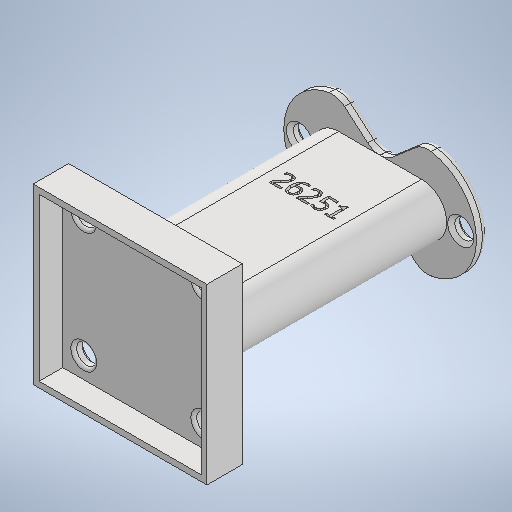
# Autodesk Inventor part: OTOSmount
Saved by Autodesk Inventor 2025.2 (Build 292293000, 293)
## iProperties
Created: 2025-01-03
Part Number: OTOSmount
Material: Generic
Document SubType Name: Modeling
Designer: dcfam
Density: 1 g/cm^3
Appearance: Default
Author: dcfam
Autodesk Inventor part; units mm, degrees
ref_plane "YZ Plane" through (0, 0, 0) normal (1, 0, 0) x (0, 1, 0)
ref_plane "XZ Plane" through (0, 0, 0) normal (0, 1, 0) x (-1, 0, 0)
ref_plane "XY Plane" through (0, 0, 0) normal (0, 0, 1) x (1, 0, 0)
sketch "Sketch1" plane through (0, 0, 0) normal (0, 0, 1) x (1, 0, 0)
  line L0 (-12.7, -12.7) -> (12.7, -12.7) construction
  line L1 (12.7, -12.7) -> (12.7, 12.7) construction
  line L2 (12.7, 12.7) -> (-12.7, 12.7) construction
  line L3 (-12.7, 12.7) -> (-12.7, -12.7) construction
  line L4 (-12.7, -12.7) -> (12.7, 12.7) construction
  line L5 (12.7, -12.7) -> (-12.7, 12.7) construction
  line L6 (14.7, -14.7) -> (-14.7, -14.7)
  line L7 (-14.7, -14.7) -> (-14.7, 14.7)
  line L8 (-14.7, 14.7) -> (14.7, 14.7)
  line L9 (14.7, 14.7) -> (14.7, -14.7)
  point P0 (0, 0)
  dimension "d0" = 25.4
  dimension "d1" = 25.4
  dimension "d2" = 2
  constraints: 20 end point, 4 parallel, 2 midpoint, 2 perpendicular, 1 horizontal, 3 other
  measures "d0" distance of L2.end L1.end
  measures "d1" distance of L1.end L0.end
  measures "d2" distance between parallel lines of L0 L6
extrude "Extrusion1" add sketch "Sketch1" along normal blind 2
sketch "Sketch2" plane through (0, 0, 2) normal (0, 0, 1) x (1, 0, 0)
  line L0 (-12.7, -12.7) -> (12.7, -12.7) construction
  line L1 (12.7, -12.7) -> (12.7, 12.7) construction
  line L2 (12.7, 12.7) -> (-12.7, 12.7) construction
  line L3 (-12.7, 12.7) -> (-12.7, -12.7) construction
  line L4 (-12.7, -12.7) -> (12.7, 12.7) construction
  line L5 (12.7, -12.7) -> (-12.7, 12.7) construction
  circle A0 centre (-10.16, 10.16) radius 1.675
  line L6 (0, 12.7) -> (0, -12.7) construction
  line L7 (-12.7, 0) -> (12.7, 0) construction
  circle A1 centre (10.16, 10.16) radius 1.675
  circle A2 centre (-10.16, -10.16) radius 1.675
  circle A3 centre (10.16, -10.16) radius 1.675
  point P0 (0, 0)
  dimension "d5" = 25.4
  dimension "d6" = 25.4
  dimension "d7" = 3.35
  dimension "d8" = 2.54
  dimension "d9" = 2.54
  constraints: 16 end point, 6 midpoint, 4 centre point, 3 symmetric about line, 2 parallel, 1 horizontal, 1 perpendicular, 3 other
  measures "d5" distance of L2.end L1.end
  measures "d6" distance of L1.end L0.end
  measures "d7" diameter of A0
  measures "d8" distance from line of L3 A0.centre
  measures "d9" distance from line of L2 A0.centre
extrude "Extrusion2" cut sketch "Sketch2" against normal blind 100
sketch "Sketch4" plane through (0, 0, 0) normal (0, 0, -1) x (-1, 0, 0)
  line L0 (-14.7, 14.7) -> (14.7, 14.7) construction
  line L1 (0, 14.7) -> (0, -14.7) construction
  line L2 (14.7, -14.7) -> (-14.7, -14.7) construction
  line L3 (-14.7, -14.7) -> (-14.7, 14.7) construction
  line L4 (-14.7, 0) -> (14.7, 0) construction
  line L5 (14.7, 14.7) -> (14.7, -14.7) construction
  line L6 (-12.7, -12.7) -> (12.7, -12.7) construction
  line L7 (12.7, -12.7) -> (12.7, 12.7) construction
  line L8 (12.7, 12.7) -> (-12.7, 12.7) construction
  line L9 (-12.7, 12.7) -> (-12.7, -12.7) construction
  line L10 (-12.7, -12.7) -> (12.7, 12.7) construction
  line L11 (12.7, -12.7) -> (-12.7, 12.7) construction
  line L12 (-7.021, 0) -> (7.021, 0) construction
  line L13 (-7.021, -4.254) -> (7.021, -4.254)
  line L14 (7.021, 4.254) -> (-7.021, 4.254)
  arc A0 (-7.021, 4.254) -> (-7.021, -4.254) centre (-7.021, 0) ccw
  arc A1 (7.021, -4.254) -> (7.021, 4.254) centre (7.021, 0) ccw
  point P0 (0, 0)
  dimension "d12" = 25.4
  dimension "d13" = 25.4
  constraints: 24 end point, 7 midpoint, 4 point on circle, 4 tangent, 3 parallel, 2 centre point, 1 horizontal, 1 perpendicular, 1 point on line
  measures "d12" distance of L8.end L7.end
  measures "d13" distance of L7.end L6.end
extrude "Extrusion3" add sketch "Sketch4" along normal blind 40
sketch "Sketch5" plane through (0, 0, -40) normal (0, 0, -1) x (-1, 0, 0)
  arc A0 (-7.021, 4.254) -> (-7.021, -4.254) centre (-7.021, 0) ccw projected
  arc A1 (7.021, -4.254) -> (7.021, 4.254) centre (7.021, 0) ccw projected
  arc A2 (7.021, -4.254) -> (7.021, 4.254) centre (7.021, 0) ccw projected
  line L0 (7.021, 4.254) -> (-7.021, 4.254) projected
  arc A3 (-7.021, 4.254) -> (-7.021, -4.254) centre (-7.021, 0) ccw projected
  line L1 (-7.021, -4.254) -> (7.021, -4.254) projected
  arc A4 (7.021, -9.254) -> (7.021, 9.254) centre (7.021, 0) ccw
  arc A5 (-7.021, 9.254) -> (-7.021, -9.254) centre (-7.021, 0) ccw
  circle A6 centre (13.6439, 0) radius 1.6
  line L2 (0, 9.254) -> (0, -9.254) construction
  circle A7 centre (-13.6439, 0) radius 1.6
  line L3 (-16.275, 0) -> (16.275, 0) construction
  line L4 (-7.021, -9.254) -> (-1.1973, -4.254)
  line L5 (-7.021, 9.254) -> (-1.1973, 4.254)
  line L6 (7.021, -9.254) -> (1.1973, -4.254)
  line L7 (7.021, 9.254) -> (1.1973, 4.254)
  point P0 (0, 0)
  point P1 (-1.1973, 4.254)
  point P2 (1.1973, 4.254)
  point P3 (1.1973, -4.254)
  dimension "d17" = 3.2
  constraints: 12 end point, 6 point on circle, 4 centre point, 4 symmetric about line, 1 point on line, 1 other
  measures "d17" diameter of A6
extrude "Extrusion4" add sketch "Sketch5" against normal blind 2
fillet "Fillet1" radius 3.175 8 edges at (-7.021, -9.254, -39) (7.021, -9.254, -39) (7.021, 9.254, -39) (-7.021, 9.254, -39) (1.1973, 4.254, -39) (-1.1973, 4.254, -39) (-1.1973, -4.254, -39) (1.1973, -4.254, -39)
chamfer "Chamfer1" distance 0.6 angle 45 4 edges at (-12.0439, 0, -38) (-12.0439, 0, -40) (15.2439, 0, -38) (15.2439, 0, -40)
fillet "Fillet2" radius 3.175 4 edges at (11.275, 0, 0) (0, 4.254, 0) (-11.275, 0, 0) (0, -4.254, 0)
chamfer "Chamfer2" distance 0.6 angle 45 4 edges at (-11.835, -10.16, 0) (8.485, -10.16, 0) (-11.835, 10.16, 0) (8.485, 10.16, 0)
sketch "Sketch7" plane through (0, 0, 2) normal (0, 0, 1) x (1, 0, 0)
  circle A0 centre (-10.16, 10.16) radius 1.675 projected
  circle A1 centre (10.16, -10.16) radius 1.675 projected
  circle A2 centre (-10.16, -10.16) radius 1.675 projected
  circle A3 centre (10.16, 10.16) radius 1.675 projected
  line L0 (14.7, 14.7) -> (-14.7, 14.7) projected
  line L1 (-14.7, 14.7) -> (-14.7, -14.7) projected
  line L2 (-14.7, -14.7) -> (14.7, -14.7) projected
  line L3 (14.7, -14.7) -> (14.7, 14.7) projected
  line L4 (12.7, 12.7) -> (-12.7, 12.7) construction
  line L5 (-12.7, 12.7) -> (-12.7, -12.7) construction
  line L6 (-12.7, -12.7) -> (12.7, -12.7) construction
  line L7 (12.7, -12.7) -> (12.7, 12.7) construction
  line L8 (12.7, 12.7) -> (-12.7, -12.7) construction
  line L9 (-12.7, 12.7) -> (12.7, -12.7) construction
  line L10 (13.7, -13.7) -> (-13.7, -13.7)
  line L11 (-13.7, -13.7) -> (-13.7, 13.7)
  line L12 (-13.7, 13.7) -> (13.7, 13.7)
  line L13 (13.7, 13.7) -> (13.7, -13.7)
  point P0 (0, 0)
  dimension "d28" = 25.4
  dimension "d29" = 25.4
  dimension "d30" = 1
  constraints: 20 end point, 2 midpoint, 2 parallel, 1 horizontal, 1 perpendicular, 3 other
  measures "d28" distance of L6.end L5.end
  measures "d29" distance of L5.end L4.end
  measures "d30" distance between parallel lines of L2 L10
extrude "Extrusion5" add sketch "Sketch7" along normal blind 4 contours L3 L2 L1 L0
sketch "Sketch9" plane through (1.1973, 4.254, -38) normal (0, 1, 0) x (1, 0, 0)
  line L0 (-6.838, -10.2364) -> (4.4434, -10.2364) construction
  line L1 (4.4434, -10.2364) -> (4.4434, -14.3898) construction
  line L2 (4.4434, -14.3898) -> (-6.838, -14.3898) construction
  line L3 (-6.838, -14.3898) -> (-6.838, -10.2364) construction
  line L4 (-6.838, -10.2364) -> (4.4434, -14.3898)
  line L5 (4.4434, -10.2364) -> (-6.838, -14.3898)
  line L6 (5.8237, -34.825) -> (-8.2183, -34.825) construction
  line L7 (5.8237, -34.825) -> (5.8237, 0) construction
  line L8 (5.8237, 0) -> (-1.176, 0) construction
  line L9 (-1.2186, 2) -> (-1.176, 2) construction
  line L10 (-1.2186, 0) -> (-8.2183, 0) construction
  line L11 (-8.2183, -34.825) -> (-8.2183, 0) construction
  line L12 (-1.1973, 2) -> (-1.1973, -34.825) construction
  line L13 (-1.176, 2) -> (-1.176, 0) projected
  line L14 (-1.2186, 0) -> (-1.2186, 2) projected
  line L15 (-4.736, -13.3487) -> (-6.6157, -13.3487)
  line L16 (-6.6157, -13.3487) -> (-6.6157, -12.9164)
  spline S0 degree 2 poles (-6.6157, -12.9164) (-6.4132, -12.7262) (-6.0525, -12.373) (-5.8796, -12.1828) knots 0 0 0 1 2 2 2
  spline S1 degree 2 poles (-5.8796, -12.1828) (-5.5314, -11.8) (-5.277, -11.3405) (-5.277, -11.096) knots 0 0 0 1 2 2 2
  spline S2 degree 2 poles (-5.277, -11.096) (-5.277, -10.9676) (-5.356, -10.7749) (-5.4276, -10.7132) knots 0 0 0 1 2 2 2
  spline S3 degree 2 poles (-5.4276, -10.7132) (-5.4993, -10.6514) (-5.687, -10.5897) (-5.8006, -10.5897) knots 0 0 0 1 2 2 2
  spline S4 degree 2 poles (-5.8006, -10.5897) (-5.9093, -10.5897) (-6.1316, -10.644) (-6.2329, -10.686) knots 0 0 0 1 2 2 2
  spline S5 degree 2 poles (-6.2329, -10.686) (-6.3193, -10.7206) (-6.4799, -10.8194) (-6.5293, -10.8539) knots 0 0 0 1 2 2 2
  line L17 (-6.5293, -10.8539) -> (-6.5515, -10.8539)
  line L18 (-6.5515, -10.8539) -> (-6.5515, -10.4192)
  spline S6 degree 2 poles (-6.5515, -10.4192) (-6.4255, -10.3575) (-5.9735, -10.2364) (-5.771, -10.2364) knots 0 0 0 1 2 2 2
  spline S7 degree 2 poles (-5.771, -10.2364) (-5.3436, -10.2364) (-4.862, -10.6885) (-4.862, -11.0738) knots 0 0 0 1 2 2 2
  spline S8 degree 2 poles (-4.862, -11.0738) (-4.862, -11.2541) (-4.946, -11.5554) (-5.0201, -11.6839) knots 0 0 0 1 2 2 2
  spline S9 degree 2 poles (-5.0201, -11.6839) (-5.0942, -11.8172) (-5.3091, -12.0791) (-5.4276, -12.205) knots 0 0 0 1 2 2 2
  spline S10 degree 2 poles (-5.4276, -12.205) (-5.6203, -12.415) (-6.0921, -12.8645) (-6.2329, -12.9954) knots 0 0 0 1 2 2 2
  line L19 (-6.2329, -12.9954) -> (-4.736, -12.9954)
  line L20 (-4.736, -12.9954) -> (-4.736, -13.3487)
  spline S11 degree 2 poles (-2.4019, -12.3607) (-2.4019, -12.5953) (-2.5575, -12.993) (-2.6884, -13.1264) knots 0 0 0 1 2 2 2
  spline S12 degree 2 poles (-2.6884, -13.1264) (-2.8242, -13.2671) (-3.1651, -13.4129) (-3.3701, -13.4129) knots 0 0 0 1 2 2 2
  spline S13 degree 2 poles (-3.3701, -13.4129) (-3.5751, -13.4129) (-3.9135, -13.2746) (-4.0419, -13.1362) knots 0 0 0 1 2 2 2
  spline S14 degree 2 poles (-4.0419, -13.1362) (-4.2, -12.9707) (-4.3779, -12.415) (-4.3779, -12.0099) knots 0 0 0 1 2 2 2
  spline S15 degree 2 poles (-4.3779, -12.0099) (-4.3779, -11.6122) (-4.2148, -10.9725) (-4.0444, -10.7354) knots 0 0 0 1 2 2 2
  spline S16 degree 2 poles (-4.0444, -10.7354) (-3.8789, -10.5032) (-3.3553, -10.2438) (-3.0119, -10.2438) knots 0 0 0 1 2 2 2
  spline S17 degree 2 poles (-3.0119, -10.2438) (-2.9107, -10.2438) (-2.7328, -10.2636) (-2.6661, -10.2858) knots 0 0 0 1 2 2 2
  line L21 (-2.6661, -10.2858) -> (-2.6661, -10.6786)
  line L22 (-2.6661, -10.6786) -> (-2.6834, -10.6786)
  spline S18 degree 2 poles (-2.6834, -10.6786) (-2.7402, -10.6489) (-2.9477, -10.5971) (-3.0663, -10.5971) knots 0 0 0 1 2 2 2
  spline S19 degree 2 poles (-3.0663, -10.5971) (-3.4467, -10.5971) (-3.9135, -11.1108) (-3.958, -11.6147) knots 0 0 0 1 2 2 2
  spline S20 degree 2 poles (-3.958, -11.6147) (-3.8122, -11.5134) (-3.506, -11.4023) (-3.3232, -11.4023) knots 0 0 0 1 2 2 2
  spline S21 degree 2 poles (-3.3232, -11.4023) (-3.1453, -11.4023) (-2.8786, -11.4739) (-2.7328, -11.5826) knots 0 0 0 1 2 2 2
  spline S22 degree 2 poles (-2.7328, -11.5826) (-2.5649, -11.7086) (-2.4019, -12.0988) (-2.4019, -12.3607) knots 0 0 0 1 2 2 2
  spline S23 degree 2 poles (-2.8168, -12.3779) (-2.8168, -12.1902) (-2.9156, -11.9358) (-3.0243, -11.8469) knots 0 0 0 1 2 2 2
  spline S24 degree 2 poles (-3.0243, -11.8469) (-3.1058, -11.7827) (-3.3084, -11.7407) (-3.4146, -11.7407) knots 0 0 0 1 2 2 2
  spline S25 degree 2 poles (-3.4146, -11.7407) (-3.5578, -11.7407) (-3.8271, -11.8271) (-3.958, -11.9086) knots 0 0 0 1 2 2 2
  spline S26 degree 2 poles (-3.958, -11.9086) (-3.9604, -11.9531) (-3.9654, -12.0371) (-3.9654, -12.1013) knots 0 0 0 1 2 2 2
  spline S27 degree 2 poles (-3.9654, -12.1013) (-3.9654, -12.4175) (-3.8419, -12.8053) (-3.748, -12.9065) knots 0 0 0 1 2 2 2
  spline S28 degree 2 poles (-3.748, -12.9065) (-3.6616, -13.0029) (-3.4738, -13.0794) (-3.3676, -13.0794) knots 0 0 0 1 2 2 2
  spline S29 degree 2 poles (-3.3676, -13.0794) (-3.1206, -13.0794) (-2.8168, -12.7287) (-2.8168, -12.3779) knots 0 0 0 1 2 2 2
  line L23 (-0.1616, -13.3487) -> (-2.0412, -13.3487)
  line L24 (-2.0412, -13.3487) -> (-2.0412, -12.9164)
  spline S30 degree 2 poles (-2.0412, -12.9164) (-1.8387, -12.7262) (-1.4781, -12.373) (-1.3052, -12.1828) knots 0 0 0 1 2 2 2
  spline S31 degree 2 poles (-1.3052, -12.1828) (-0.9569, -11.8) (-0.7025, -11.3405) (-0.7025, -11.096) knots 0 0 0 1 2 2 2
  spline S32 degree 2 poles (-0.7025, -11.096) (-0.7025, -10.9676) (-0.7815, -10.7749) (-0.8532, -10.7132) knots 0 0 0 1 2 2 2
  spline S33 degree 2 poles (-0.8532, -10.7132) (-0.9248, -10.6514) (-1.1125, -10.5897) (-1.2261, -10.5897) knots 0 0 0 1 2 2 2
  spline S34 degree 2 poles (-1.2261, -10.5897) (-1.3348, -10.5897) (-1.5571, -10.644) (-1.6584, -10.686) knots 0 0 0 1 2 2 2
  spline S35 degree 2 poles (-1.6584, -10.686) (-1.7448, -10.7206) (-1.9054, -10.8194) (-1.9548, -10.8539) knots 0 0 0 1 2 2 2
  line L25 (-1.9548, -10.8539) -> (-1.977, -10.8539)
  line L26 (-1.977, -10.8539) -> (-1.977, -10.4192)
  spline S36 degree 2 poles (-1.977, -10.4192) (-1.851, -10.3575) (-1.399, -10.2364) (-1.1965, -10.2364) knots 0 0 0 1 2 2 2
  spline S37 degree 2 poles (-1.1965, -10.2364) (-0.7692, -10.2364) (-0.2875, -10.6885) (-0.2875, -11.0738) knots 0 0 0 1 2 2 2
  spline S38 degree 2 poles (-0.2875, -11.0738) (-0.2875, -11.2541) (-0.3715, -11.5554) (-0.4456, -11.6839) knots 0 0 0 1 2 2 2
  spline S39 degree 2 poles (-0.4456, -11.6839) (-0.5197, -11.8172) (-0.7346, -12.0791) (-0.8532, -12.205) knots 0 0 0 1 2 2 2
  spline S40 degree 2 poles (-0.8532, -12.205) (-1.0458, -12.415) (-1.5176, -12.8645) (-1.6584, -12.9954) knots 0 0 0 1 2 2 2
  line L27 (-1.6584, -12.9954) -> (-0.1616, -12.9954)
  line L28 (-0.1616, -12.9954) -> (-0.1616, -13.3487)
  spline S41 degree 2 poles (2.0936, -12.3804) (2.0936, -12.6002) (1.9528, -12.9757) (1.8243, -13.114) knots 0 0 0 1 2 2 2
  spline S42 degree 2 poles (1.8243, -13.114) (1.6959, -13.2523) (1.313, -13.4129) (1.0759, -13.4129) knots 0 0 0 1 2 2 2
  spline S43 degree 2 poles (1.0759, -13.4129) (0.8586, -13.4129) (0.4337, -13.3165) (0.2781, -13.24) knots 0 0 0 1 2 2 2
  line L29 (0.2781, -13.24) -> (0.2781, -12.8077)
  line L30 (0.2781, -12.8077) -> (0.3078, -12.8077)
  spline S44 degree 2 poles (0.3078, -12.8077) (0.3547, -12.8423) (0.5301, -12.9312) (0.6363, -12.9707) knots 0 0 0 1 2 2 2
  spline S45 degree 2 poles (0.6363, -12.9707) (0.7573, -13.0127) (0.9574, -13.0597) (1.0833, -13.0597) knots 0 0 0 1 2 2 2
  spline S46 degree 2 poles (1.0833, -13.0597) (1.2068, -13.0597) (1.439, -12.9707) (1.523, -12.8744) knots 0 0 0 1 2 2 2
  spline S47 degree 2 poles (1.523, -12.8744) (1.5996, -12.783) (1.6786, -12.541) (1.6786, -12.3779) knots 0 0 0 1 2 2 2
  spline S48 degree 2 poles (1.6786, -12.3779) (1.6786, -12.2149) (1.5897, -12.0074) (1.5057, -11.9383) knots 0 0 0 1 2 2 2
  spline S49 degree 2 poles (1.5057, -11.9383) (1.4193, -11.8617) (1.1624, -11.7975) (1.0068, -11.7975) knots 0 0 0 1 2 2 2
  spline S50 degree 2 poles (1.0068, -11.7975) (0.8388, -11.7975) (0.5054, -11.8494) (0.4041, -11.8716) knots 0 0 0 1 2 2 2
  line L31 (0.4041, -11.8716) -> (0.4041, -10.3007)
  line L32 (0.4041, -10.3007) -> (2.0763, -10.3007)
  line L33 (2.0763, -10.3007) -> (2.0763, -10.6588)
  line L34 (2.0763, -10.6588) -> (0.7968, -10.6588)
  line L35 (0.7968, -10.6588) -> (0.7968, -11.4714)
  spline S51 degree 2 poles (0.7968, -11.4714) (0.8709, -11.4616) (1.0142, -11.4542) (1.0735, -11.4542) knots 0 0 0 1 2 2 2
  spline S52 degree 2 poles (1.0735, -11.4542) (1.3081, -11.4542) (1.6317, -11.5307) (1.7799, -11.6443) knots 0 0 0 1 2 2 2
  spline S53 degree 2 poles (1.7799, -11.6443) (1.9306, -11.758) (2.0936, -12.1038) (2.0936, -12.3804) knots 0 0 0 1 2 2 2
  line L36 (4.2598, -13.3487) -> (2.7728, -13.3487)
  line L37 (2.7728, -13.3487) -> (2.7728, -13.0374)
  line L38 (2.7728, -13.0374) -> (3.3261, -13.0374)
  line L39 (3.3261, -13.0374) -> (3.3261, -10.9947)
  line L40 (3.3261, -10.9947) -> (2.7728, -10.9947)
  line L41 (2.7728, -10.9947) -> (2.7728, -10.7156)
  spline S54 degree 2 poles (2.7728, -10.7156) (3.0865, -10.7156) (3.3829, -10.5378) (3.4027, -10.2908) knots 0 0 0 1 2 2 2
  line L42 (3.4027, -10.2908) -> (3.7188, -10.2908)
  line L43 (3.7188, -10.2908) -> (3.7188, -13.0374)
  line L44 (3.7188, -13.0374) -> (4.2598, -13.0374)
  line L45 (4.2598, -13.0374) -> (4.2598, -13.3487)
  point P0 (-1.1973, -38)
  point P1 (-1.1973, -12.3131)
  constraints: 6 end point, 3 midpoint, 1 point on line, 1 vertical, 2 other
emboss "Emboss1" sketch "Sketch9" operation cut depth 0.5 direction (0, -1, 0) contours S6 S7 L4 S2 S3 S4 | L4 S4 S5 L17 L18 S6 | L4 S7 S8 S9 S10 L19 L20 L15 L16 S0 S1 S2 | S15 S16 S17 L21 L22 S18 S19 L4 | L4 S19 S20 S22 S11 L5 S29 S23 S24 S25 S26 S27 S28 S13 S14 S15 | S20 S21 S22 L4 | L5 S29 S11 S12 S13 | S30 S31 S32 S33 S34 S35 L25 L26 S36 S37 S38 S39 L5 L4 | L4 L5 S30 | L5 S39 S40 L4 | L4 S40 L27 L28 L23 L24 S30 L5 | L29 L30 S44 S45 S46 S47 S48 S49 S50 L31 L5 S52 S53 S41 S42 L4 | L4 S42 S43 L29 | L31 L32 L33 L34 L35 S51 S52 L5 | L43 L44 L45 L36 L37 L38 L39 L40 L41 L5 | L5 L41 S54 L42 L43
fillet "Fillet5" radius 0.5 4 edges at (8.485, 10.16, 2) (-11.835, 10.16, 2) (-11.835, -10.16, 2) (8.485, -10.16, 2)
fillet "Fillet6" radius 1 12 edges at (0, 4.254, -40) (0, -4.254, -40) (-4.0543, 6.7069, -40) (-1.1241, 4.4517, -40) (1.1241, 4.4517, -40) (4.0543, 6.7069, -40) (16.275, 0, -40) (4.0543, -6.7069, -40) (1.1241, -4.4517, -40) (-1.1241, -4.4517, -40) (-4.0543, -6.7069, -40) (-16.275, 0, -40)
body "Solid1"
